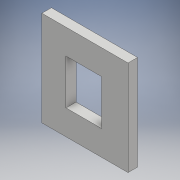
# Autodesk Inventor part: TapaFrontal
Saved by Autodesk Inventor 2017 (Build 210142000, 142)
## iProperties
Created: 2021-02-12
Part Number: TapaFrontal
Material: Generic
Document SubType Name: Modeling
Designer: USUARIO
Density: 1 g/cm^3
Appearance: Default
Author: USUARIO
Autodesk Inventor part; units mm, degrees
ref_plane "YZ Plane" through (0, 0, 0) normal (1, 0, 0) x (0, 1, 0)
ref_plane "XZ Plane" through (0, 0, 0) normal (0, 1, 0) x (-1, 0, 0)
ref_plane "XY Plane" through (0, 0, 0) normal (0, 0, 1) x (1, 0, 0)
sketch "Sketch1" plane through (0, 0, 0) normal (0, 1, 0) x (-1, 0, 0)
  line L0 (0, 0) -> (460, 0)
  line L1 (460, 0) -> (460, -507)
  line L2 (460, -507) -> (0, -507)
  line L3 (0, -507) -> (0, 0)
  line L4 (331.3, -133.5) -> (141.3, -133.5)
  line L5 (141.3, -133.5) -> (141.3, -373.5)
  line L6 (141.3, -373.5) -> (331.3, -373.5)
  line L7 (331.3, -373.5) -> (331.3, -133.5)
  dimension "d0" = 460
  dimension "d1" = 507
  dimension "d2" = 190
  dimension "d3" = 240
  dimension "d4" = 133.5
  dimension "d5" = 141.3
  constraints: 16 end point, 4 parallel, 2 horizontal, 2 perpendicular
  measures "d0" distance of L1.end L2.end
  measures "d1" distance of L0.end L1.end
  measures "d2" distance of L6.end L5.end
  measures "d3" distance of L5.end L4.end
  measures "d4" distance between parallel lines of L2 L6
  measures "d5" distance between parallel lines of L3 L5
extrude "Extrusion1" add sketch "Sketch1" along normal blind 50.8
sketch "Sketch5" plane through (0, 50.8, 0) normal (0, 1, 0) x (1, 0, 0)
  line L0 (-406, 54) -> (-54, 54)
  line L1 (-54, 54) -> (-54, 453)
  line L2 (-54, 453) -> (-406, 453)
  line L3 (-406, 453) -> (-406, 54)
  line L4 (-460, 0) -> (0, 0) projected
  line L5 (-460, 507) -> (-460, 0) projected
  line L6 (-331.3, 133.5) -> (-141.3, 133.5) projected
  line L7 (-141.3, 373.5) -> (-331.3, 373.5) projected
  line L8 (-331.3, 133.5) -> (-141.3, 133.5)
  line L9 (-141.3, 133.5) -> (-141.3, 373.5)
  line L10 (-141.3, 373.5) -> (-331.3, 373.5)
  line L11 (-331.3, 373.5) -> (-331.3, 133.5)
  dimension "d14" = 352
  dimension "d15" = 399
  dimension "d16" = 54
  dimension "d17" = 54
  constraints: 16 end point, 4 parallel, 2 horizontal, 2 perpendicular
  measures "d14" distance of L2.end L1.end
  measures "d15" distance of L1.end L0.end
  measures "d16" distance between parallel lines of L0 L4
  measures "d17" distance between parallel lines of L5 L3
extrude "Extrusion2" add sketch "Sketch5" along normal blind 3
body "Solid1"
